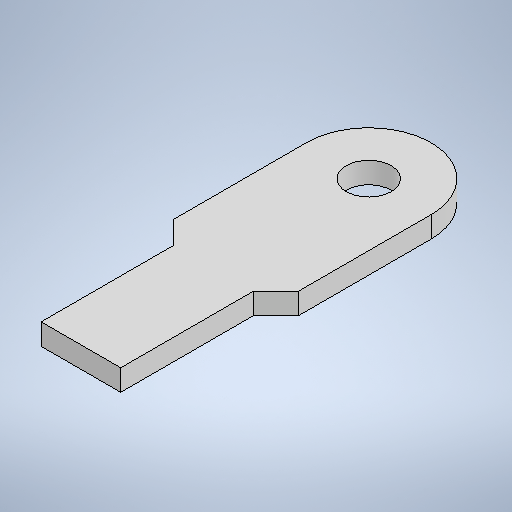
# Autodesk Inventor part: PNS-073 stretch tear
Saved by Autodesk Inventor 2025 (Build 290162010, 162A)
## iProperties
Created: 2025-03-26
Part Number: PNS-073 stretch tear
Material: Stainless Steel
Description: DIE16(5)|\ 90°|corrY -___°|X_____|bom___
Document SubType Name: Sheet Metal
Designer: user
Stock Number: МОО 305 шпангоут борт
Mass: 308.336 g
Surface Area: 126.857 cm^2
Volume: 38.5419 cm^3
Density: 8 g/cm^3
Sheet Metal Rule: AISI304 2mm Die16
Sheet Metal Width: 47,000 mm
Sheet Metal Length: 132,000 mm
Sheet Metal Area: 6204,000 mm^2
Appearance: Default
Flat Pattern Width: 4.7 cm
Flat Pattern Length: 13.2 cm
Flat Pattern Area: 62.04 cm^2
Author: admin
Autodesk Inventor part; units mm, degrees
ref_plane "YZ Plane" through (0, 0, 0) normal (1, 0, 0) x (0, 1, 0)
ref_plane "XZ Plane" through (0, 0, 0) normal (0, 1, 0) x (-1, 0, 0)
ref_plane "XY Plane" through (0, 0, 0) normal (0, 0, 1) x (1, 0, 0)
sketch "Sketch1" plane through (0, 0, 0) normal (0, 0, 1) x (1, 0, 0)
  circle A0 centre (0, 0) radius 8.5
  arc A1 (23.5, 0) -> (-23.5, 0) centre (0, 0) ccw
  line L0 (-23.5, 0) -> (-23.5, -50)
  line L1 (-23.5, -50) -> (-15, -58.5)
  line L2 (-15, -58.5) -> (-15, -108.5)
  line L3 (-15, -108.5) -> (15, -108.5)
  line L4 (15, -108.5) -> (15, -58.5)
  line L5 (15, -58.5) -> (23.5, -50)
  line L6 (23.5, -50) -> (23.5, 0)
  line L7 (0, 0) -> (0, -108.5) construction
  dimension "d162" = 17
  dimension "d163" = 15
  dimension "d164" = 50
  dimension "d165" = 45
  dimension "d166" = 50
  dimension "d167" = 30
  measures "d162" diameter of A0
  measures "d163" radial gap between concentric circles of A0 A1
  measures "d164" distance of L0.start L0.end
  measures "d165" angle of L0 L1
  measures "d166" distance of L1.end L2.end
  measures "d167" distance of L2.end L3.end
extrude "Plate5" add sketch "Sketch1" along normal blind 8
body "Solid3"
